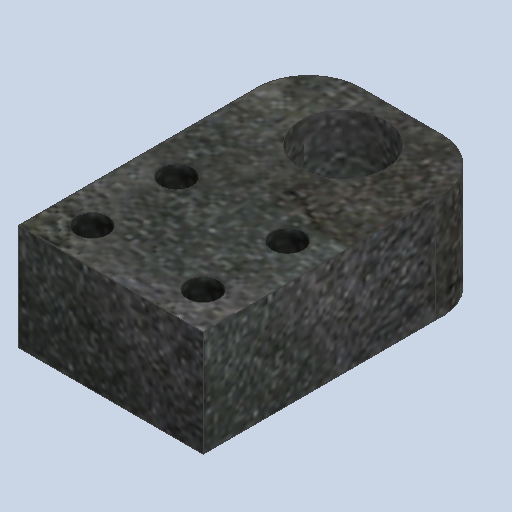
# Autodesk Inventor part: spindel sockel
Saved by Autodesk Inventor 2023.2 (Build 272271000, 271)
## iProperties
Created: 2023-02-05
Part Number: spindel sockel
Material: Steel
Document SubType Name: Modeling
Designer: Ayush
Density: 7.85 g/cm^3
Appearance: Plate
Author: Ayush
Autodesk Inventor part; units mm, degrees
ref_plane "YZ Plane" through (0, 0, 0) normal (1, 0, 0) x (0, 1, 0)
ref_plane "XZ Plane" through (0, 0, 0) normal (0, 1, 0) x (-1, 0, 0)
ref_plane "XY Plane" through (0, 0, 0) normal (0, 0, 1) x (1, 0, 0)
sketch "Sketch1" plane through (0, 0, 0) normal (0, 1, 0) x (-1, 0, 0)
  line L0 (-17.5, 27.5) -> (17.5, 27.5)
  line L1 (-17.5, 27.5) -> (17.5, -27.5) construction
  line L2 (17.5, 27.5) -> (-17.5, -27.5) construction
  circle A0 centre (10.5, 4.5) radius 5.5
  circle A1 centre (-10.5, 4.5) radius 5.5
  circle A2 centre (-10.5, 20.5) radius 5.5
  circle A3 centre (10.5, 20.5) radius 5.5
  line L3 (17.5, 27.5) -> (17.5, -16.5)
  line L4 (-17.5, 27.5) -> (-17.5, -16.5)
  circle A4 centre (0, -16.5) radius 8
  line L5 (8, -27.5) -> (-8, -27.5)
  arc A5 (8, -27.5) -> (17.5, -16.5) centre (7.5511, -17.5101) ccw
  arc A6 (-17.5, -16.5) -> (-8, -27.5) centre (-7.5511, -17.5101) ccw
  point P0 (0, 0)
  point P1 (0, 27.5)
  dimension "d0" = 35
  dimension "d1" = 55
  dimension "d5" = 11
  dimension "d7" = 11
  dimension "d9" = 11
  dimension "d11" = 11
  dimension "d13" = 7
  dimension "d15" = 23
  dimension "d16" = 21
  dimension "d17" = 10.5
  dimension "d18" = 44
  dimension "d19" = 16
  dimension "d20" = 44
  dimension "d25" = 10
  dimension "d26" = 10
  constraints: 12 end point, 7 centre point, 4 point on circle, 3 midpoint, 2 horizontal, 2 horizontal alignment, 2 vertical, 2 vertical alignment
  measures "d0" distance of L1.end L2.end
  measures "d1" distance of L0.end L1.end
  measures "d5" diameter of A0
  measures "d7" diameter of A1
  measures "d9" diameter of A2
  measures "d11" diameter of A3
  measures "d13" distance from line of A3.centre L0
  measures "d15" distance from line of A0.centre L0
  measures "d16" distance of A1.centre A0.centre
  measures "d17" horizontal distance of point (0, 27.5) A0.centre
  measures "d18" distance of L0.end L3.end
  measures "d19" diameter of A4
  measures "d20" distance from line of A4.centre L0
  measures "d25" radius of A5
  measures "d26" radius of A6
extrude "Extrusion1" add sketch "Sketch1" along normal blind 7
sketch "Sketch2" plane through (0, 7, 0) normal (0, 1, 0) x (1, 0, 0)
  line L0 (-17.5, 16.5) -> (-17.5, -27.5) projected
  line L1 (-17.5, -27.5) -> (-17.5, 16.5)
  line L2 (8, 27.5) -> (-8, 27.5) projected
  line L3 (-8, 27.5) -> (8, 27.5)
  line L4 (17.5, -27.5) -> (17.5, 16.5) projected
  line L5 (17.5, 16.5) -> (17.5, -27.5)
  line L6 (-17.5, -27.5) -> (17.5, -27.5) projected
  line L7 (17.5, -27.5) -> (-17.5, -27.5)
  circle A0 centre (0, 16.5) radius 8
  circle A1 centre (-10.5, -4.5) radius 3
  circle A2 centre (10.5, -4.5) radius 3
  circle A3 centre (10.5, -20.5) radius 3
  circle A4 centre (-10.5, -20.5) radius 3
  arc A5 (-8, 27.5) -> (-17.5, 16.5) centre (-7.5511, 17.5101) ccw projected
  arc A6 (-8, 27.5) -> (-17.5, 16.5) centre (-7.5511, 17.5101) ccw
  arc A7 (17.5, 16.5) -> (8, 27.5) centre (7.5511, 17.5101) ccw
  point P0 (0, 0)
  point P1 (0, -27.5)
  dimension "d29" = 16
  dimension "d30" = 6
  dimension "d31" = 6
  dimension "d32" = 6
  dimension "d33" = 6
  dimension "d34" = 7
  dimension "d35" = 23
  dimension "d36" = 21
  dimension "d37" = 10.5
  constraints: 8 end point, 7 centre point, 4 collinear, 4 point on circle, 2 horizontal alignment, 2 vertical alignment, 1 midpoint
  measures "d29" diameter of A0
  measures "d30" diameter of A1
  measures "d31" diameter of A2
  measures "d32" diameter of A3
  measures "d33" diameter of A4
  measures "d34" distance from line of A4.centre L6
  measures "d35" distance from line of A1.centre L6
  measures "d36" distance of A2.centre A1.centre
  measures "d37" horizontal distance of point (0, -27.5) A1.centre
extrude "Extrusion2" add sketch "Sketch2" along normal blind 13
body "Solid1"
